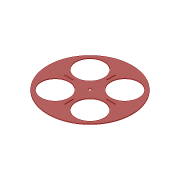
# Autodesk Inventor part: Plate
Saved by Autodesk Inventor 2018 (Build 220112000, 112)
## iProperties
Created: 2017-11-16
Part Number: Plate
Material: Aluminum 6061
Document SubType Name: Modeling
Designer: Udara Wanasinghe
Density: 2.7 g/cm^3
Appearance: Aluminum - Flat(1)
Mass: 206.366 g
Surface Area: 813.645 cm^2
Volume: 76.4318 cm^3
Author: Udara Wanasinghe
Autodesk Inventor part; units mm, degrees
ref_plane "YZ Plane" through (0, 0, 0) normal (1, 0, 0) x (0, 1, 0)
ref_plane "XZ Plane" through (0, 0, 0) normal (0, 1, 0) x (-1, 0, 0)
ref_plane "XY Plane" through (0, 0, 0) normal (0, 0, 1) x (1, 0, 0)
sketch "Sketch1" plane through (0, 0, 0) normal (0, 1, 0) x (-1, 0, 0)
  circle A0 centre (0, 0) radius 150
  dimension "d0" = 300
  constraints: 1 centre point, 1 coincident
  measures "d0" diameter of A0
extrude "Extrusion1" add sketch "Sketch1" along normal blind 2
sketch "Sketch2" plane through (0, 2, 0) normal (0, 1, 0) x (1, 0, 0)
  circle A0 centre (62.132, 62.132) radius 50
  circle A1 centre (0, 0) radius 150 construction
  line L0 (0, 150) -> (0, -150) construction
  line L1 (150, 0) -> (-150, 0) construction
  line L2 (62.132, 62.132) -> (0, 62.132) construction
  line L3 (62.132, 62.132) -> (62.132, 0) construction
  line L4 (62.132, 62.132) -> (106.066, 106.066) construction
  dimension "d3" = 100
  dimension "d26" = 62.132
  constraints: 10 end point, 5 point on circle, 3 midpoint, 3 perpendicular, 2 equal length, 2 point on line, 1 centre point, 1 vertical, 1 other
  measures "d3" diameter of A0
  measures "d26" distance of L2.start L2.end
extrude "Extrusion2" cut sketch "Sketch2" against normal through all
pattern_circular "Circular Pattern1" count 4 over 360 about axis through (0, -10, 0) along (0, 1, 0) of "Extrusion2"
sketch "Sketch3" plane through (0, 2, 0) normal (0, 1, 0) x (1, 0, 0)
  circle A0 centre (0, 0) radius 5
  dimension "d9" = 10
  constraints: 1 centre point, 1 coincident
  measures "d9" diameter of A0
extrude "Extrusion3" cut sketch "Sketch3" against normal through all
sketch "Sketch5" plane through (0, 2, 0) normal (0, 1, 0) x (1, 0, 0)
  circle A0 centre (0, 0) radius 5 construction
  line L0 (0, 0) -> (-150, 0) construction
  arc A1 (-150, 0) -> (-150, 0) centre (0, 0) ccw construction
  line L1 (-60, -1) -> (-60, 1)
  line L2 (-60, 1) -> (-90, 1)
  line L3 (-90, 1) -> (-90, -1)
  line L4 (-90, -1) -> (-60, -1)
  line L5 (-60, 0) -> (-90, 0) construction
  point P0 (-75, 0)
  dimension "d19" = 2
  dimension "d20" = 30
  constraints: 12 end point, 4 midpoint, 3 perpendicular, 1 horizontal, 1 point on circle, 1 vertical
  measures "d19" distance from line of L2 L1.start
  measures "d20" distance of L1.end L2.end
extrude "Extrusion5" cut sketch "Sketch5" against normal through all
pattern_circular "Circular Pattern3" count 4 over 360 about axis through (0, -10, 0) along (0, 1, 0) of "Extrusion5"
body "Solid1"
